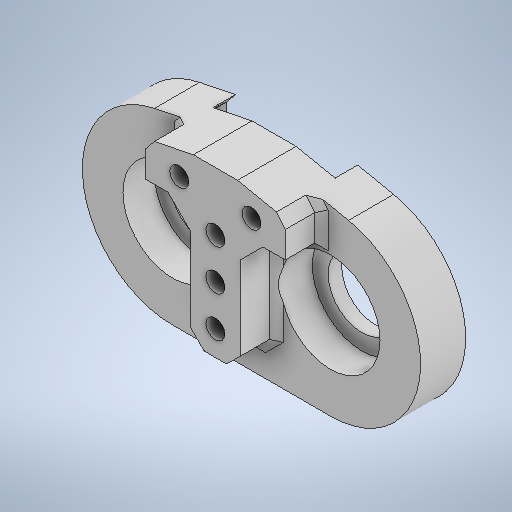
# Autodesk Inventor part: 悬臂架
Saved by Autodesk Inventor 2025.1 (Build 291241000, 241)
## iProperties
Created: 2025-08-27
Part Number: 悬臂架
Material: 常规
Document SubType Name: Modeling
Designer: Piw
Density: 1 g/cm^3
Appearance: 默认
Author: Piw
Autodesk Inventor part; units mm, degrees
ref_plane "YZ Plane" through (0, 0, 0) normal (1, 0, 0) x (0, 1, 0)
ref_plane "XZ Plane" through (0, 0, 0) normal (0, 1, 0) x (-1, 0, 0)
ref_plane "XY Plane" through (0, 0, 0) normal (0, 0, 1) x (1, 0, 0)
sketch "草图1" plane through (0, 0, 0) normal (0, 0, 1) x (1, 0, 0)
  circle A0 centre (-17.5, 0) radius 11
  line L0 (0, 60.0767) -> (0, -61.2503)
  line L1 (-58.4326, 0) -> (36.5091, 0) construction
  arc A1 (-21.5135, 19.5932) -> (-17.5, -20) centre (-17.5, 0) ccw
  line L2 (-21.5135, 19.5932) -> (0, 24)
  line L3 (-17.5, -20) -> (0, -20)
  arc A2 (2.5, 0) -> (-21.5135, 19.5932) centre (-17.5, 0) ccw construction
  arc A3 (-17.5, -20) -> (2.5, 0) centre (-17.5, 0) ccw construction
  circle A4 centre (17.5, 0) radius 11
  arc A5 (17.5, -20) -> (21.5135, 19.5932) centre (17.5, 0) ccw
  line L4 (21.5135, 19.5932) -> (0, 24)
  line L5 (17.5, -20) -> (0, -20)
  arc A6 (21.5135, 19.5932) -> (-2.5, 0) centre (17.5, 0) ccw construction
  arc A7 (-2.5, 0) -> (17.5, -20) centre (17.5, 0) ccw construction
  point P0 (0, 0)
  point P1 (58.4326, 0)
  dimension "d0" = 22
  dimension "d1" = 35
  dimension "d2" = 40
  dimension "d3" = 24
  constraints: 12 end point, 12 point on circle, 8 centre point, 6 symmetric about line, 4 point on line, 4 tangent, 3 horizontal, 2 coincident, 2 vertical, 4 other
  measures "d0" diameter of A0
  measures "d1" diameter of A0.centre L0
  measures "d2" diameter of A1
  measures "d3" distance from line of L1 L2.end
extrude "拉伸1" add sketch "草图1" along normal blind 7
sketch "草图2" plane through (0, 0, 0) normal (0, 0, -1) x (-1, 0, 0)
  arc A0 (-21.5135, 19.5932) -> (-17.5, -20) centre (-17.5, 0) ccw projected
  arc A1 (-21.5135, 19.5932) -> (-17.5, -20) centre (-17.5, 0) ccw projected
  line L0 (17.5, -20) -> (-17.5, -20) projected
  arc A2 (17.5, -20) -> (21.5135, 19.5932) centre (17.5, 0) ccw projected
  line L1 (0, 24) -> (21.5135, 19.5932) projected
  circle A3 centre (17.5, 0) radius 11 projected
  circle A4 centre (-17.5, 0) radius 11 projected
  circle A5 centre (-17.5, 0) radius 7.5
  circle A6 centre (17.5, 0) radius 7.5
  line L2 (-21.5135, 19.5932) -> (0, 24) projected
  point P0 (0, 0)
  dimension "d6" = 15
  dimension "d7" = 15
  constraints: 2 centre point, 2 coincident
  measures "d6" diameter of A5
  measures "d7" diameter of A6
extrude "拉伸2" add sketch "草图2" along normal blind 3 contours L2 L1 A2 L0 A0 | A3 | A4
chamfer "倒角1" distance 5 angle 45 1 edges at (0, 24, 2)
sketch "草图3" plane through (0, 0, 7) normal (0, 0, 1) x (1, 0, 0)
  line L0 (-5.5, 13.5) -> (5.5, 13.5) construction
  line L1 (5.5, 13.5) -> (5.5, 13) construction
  line L2 (5.5, -13.5) -> (-5.5, -13.5)
  line L3 (-5.5, -13.5) -> (-5.5, 13)
  line L4 (-5.5, 13.5) -> (5.5, -13.5) construction
  line L5 (5.5, 13.5) -> (-5.5, -13.5) construction
  line L6 (5.5, 13) -> (15.5, 13)
  line L7 (15.5, 13) -> (15.5, 20.825)
  line L8 (21.5135, 19.5932) -> (4.8983, 22.9966) projected
  line L9 (5.5, 13) -> (5.5, -13.5)
  line L10 (-4.8983, 22.9966) -> (4.8983, 22.9966) projected
  line L11 (0, 34.3003) -> (0, -25.0257) construction
  line L12 (-5.5, 13) -> (-15.5, 13)
  line L13 (-15.5, 13) -> (-15.5, 20.825)
  line L14 (-5.5, 13) -> (-5.5, 13.5) construction
  line L15 (-4.8983, 22.9966) -> (-21.5135, 19.5932) projected
  point P0 (0, 0)
  dimension "d13" = 11
  dimension "d14" = 27
  dimension "d18" = 13
  dimension "d19" = 10
  constraints: 26 end point, 5 parallel, 3 symmetric about line, 3 vertical, 2 horizontal, 2 midpoint, 2 perpendicular, 1 point on line
  measures "d13" distance of L2.start L2.end
  measures "d14" distance of L2.end L0.start
  measures "d18" distance from line of point (0, 0) L6
  measures "d19" distance between parallel lines of L1 L7
extrude "拉伸3" add sketch "草图3" along normal blind 8
chamfer "倒角2" distance 5 angle 45 2 edges at (-5.5, 13, 11) (5.5, 13, 11)
chamfer "倒角3" distance 3 angle 45 2 edges at (-5.5, -13.5, 11) (5.5, -13.5, 11)
chamfer "倒角4" distance 2 angle 45 2 edges at (15.5, 20.825, 11) (-15.5, 20.825, 11)
sketch "草图6" plane through (0, 0, 15) normal (0, 0, 1) x (1, 0, 0)
  circle A0 centre (0, -8) radius 2.1
  line L0 (0, 37.234) -> (0, -34.1574)
  circle A1 centre (8, 17.2575) radius 2.1
  line L1 (-19.2102, 22.8312) -> (5.0899, 17.8536) construction
  line L2 (13.5407, 21.2263) -> (4.8983, 22.9966) projected
  line L3 (-2.5, -13.5) -> (2.5, -13.5) projected
  circle A2 centre (-8, 17.2575) radius 2.1
  circle A3 centre (0, 1) radius 2.1
  circle A4 centre (0, 10) radius 2.1
  point P0 (0, 0)
  dimension "d48" = 4.2
  dimension "d49" = 4.2
  dimension "d50" = 5
  dimension "d51" = 16
  dimension "d53" = 8
  dimension "d77" = 4.2
  dimension "d78" = 1
  dimension "d79" = 4.2
  dimension "d80" = 9
  constraints: 5 centre point, 4 end point, 4 point on line, 2 vertical, 1 parallel, 1 symmetric about line, 1 other
  measures "d48" diameter of A0
  measures "d49" diameter of A1
  measures "d50" distance between parallel lines of L2 L1
  measures "d51" diameter of A1.centre L0
  measures "d53" distance of A0.centre point (0, 0)
  measures "d77" diameter of A3
  measures "d78" distance of point (0, 0) A3.centre
  measures "d79" diameter of A4
  measures "d80" distance of A3.centre A4.centre
extrude "拉伸5" cut sketch "草图6" against normal through all
chamfer "倒角7" distance 1.5 angle 45 13 edges at (-15.5, 15.9125, 7) (-13, 13, 7) (-8, 10.5, 7) (-5.5, -1.25, 7) (-4, -12, 7) (0, -13.5, 7) (4, -12, 7) (5.5, -1.25, 7) (8, 10.5, 7) (13, 13, 7) (15.5, 15.9125, 7) (14.5203, 20.0256, 7) (-14.5203, 20.0256, 7)
sketch "草图9" plane through (0, 0, -3) normal (0, 0, -1) x (-1, 0, 0)
  line L0 (5.5, 8) -> (5.5, -10.5) projected
  line L1 (2.5, -13.5) -> (5.5, -10.5) projected
  line L2 (2.5, -13.5) -> (-2.5, -13.5) projected
  line L3 (-5.5, -10.5) -> (-2.5, -13.5) projected
  line L4 (-5.5, -10.5) -> (-5.5, 8) projected
  line L5 (-10.5, 13) -> (-5.5, 8) projected
  line L6 (-10.5, 13) -> (-15.5, 13) projected
  line L7 (-15.5, 13) -> (-15.5, 18.825) projected
  line L8 (-13.5407, 21.2263) -> (-15.5, 18.825) projected
  line L9 (-13.5407, 21.2263) -> (-4.8983, 22.9966) projected
  line L10 (-4.8983, 22.9966) -> (4.8983, 22.9966) projected
  line L11 (4.8983, 22.9966) -> (13.5407, 21.2263) projected
  line L12 (15.5, 18.825) -> (13.5407, 21.2263) projected
  line L13 (15.5, 18.825) -> (15.5, 13) projected
  line L14 (15.5, 13) -> (10.5, 13) projected
  line L15 (5.5, 8) -> (10.5, 13) projected
  point P0 (0, 0)
extrude "拉伸7" cut sketch "草图9" against normal blind 5
